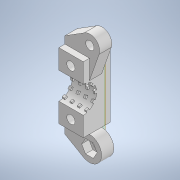
# Autodesk Inventor part: Rear Cable Clamp
Saved by Autodesk Inventor 2020 (Build 240168000, 168)
## iProperties
Created: 2019-12-14
Part Number: Rear Cable Clamp
Material: Generic
Document SubType Name: Modeling
Designer: pepd9
Density: 1 g/cm^3
Appearance: Default
Author: pepd9
Autodesk Inventor part; units mm, degrees
ref_plane "YZ Plane" through (0, 0, 0) normal (1, 0, 0) x (0, 1, 0)
ref_plane "XZ Plane" through (0, 0, 0) normal (0, 1, 0) x (-1, 0, 0)
ref_plane "XY Plane" through (0, 0, 0) normal (0, 0, 1) x (1, 0, 0)
sketch "Sketch1" plane through (0, 0, 0) normal (0, 0, 1) x (1, 0, 0)
  circle A0 centre (0, 0) radius 1.7
  circle A1 centre (0, 0) radius 5
  line L0 (0, 7) -> (0, -7) projected
  dimension "d0" = 10
  dimension "d6" = 3.4
  constraints: 2 centre point, 1 coincident
  measures "d0" diameter of A1
  measures "d6" diameter of A0
extrude "Extrusion1" add sketch "Sketch1" along normal blind 5 contours A0 L0 A1 | A0 L0 A1
sketch "Sketch2" plane through (0, 0, 5) normal (0, 0, 1) x (1, 0, 0)
  circle A0 centre (0, 0) radius 1.7 projected
  line L0 (1.5877, 2.75) -> (3.1754, 0)
  line L1 (3.1754, 0) -> (1.5877, -2.75)
  line L2 (1.5877, -2.75) -> (-1.5877, -2.75)
  line L3 (-1.5877, -2.75) -> (-3.1754, 0)
  line L4 (-3.1754, 0) -> (-1.5877, 2.75)
  line L5 (-1.5877, 2.75) -> (1.5877, 2.75)
  dimension "d3" = 5.5
  constraints: 12 end point, 1 coincident, 1 horizontal, 13 other
  measures "d3" distance between parallel lines of L2 L5
extrude "Extrusion2" cut sketch "Sketch2" against normal blind 3
sketch "Sketch3" plane through (0, 0, 0) normal (0, 0, -1) x (-1, 0, 0)
  point P0 (0, 0)
sketch "Sketch4" plane through (0, 0, 0) normal (1, 0, 0) x (0, 1, 0)
  line L0 (5, 0) -> (5, 5) projected
  line L1 (5, -3.5) -> (32, -3.5)
  line L2 (32, -3.5) -> (32, 7.5)
  line L3 (32, 7.5) -> (5, 7.5)
  line L4 (5, 7.5) -> (5, -3.5)
  circle A0 centre (18.5, 7.5) radius 5.5
  line L5 (5, 5) -> (-5, 5) projected
  point P0 (0, 0)
  point P1 (24, 7.5)
  point P2 (13, 7.5)
  dimension "d7" = 11
  dimension "d8" = 27
  dimension "d9" = 13.5
  dimension "d12" = 2.5
  dimension "d13" = 11
  constraints: 8 end point, 2 parallel, 1 centre point, 1 horizontal, 1 midpoint, 1 perpendicular, 1 point on line
  measures "d7" diameter of A0
  measures "d8" distance of L1.start L1.end
  measures "d9" distance from line of L4 A0.centre
  measures "d12" distance between parallel lines of L5 L3
  measures "d13" distance from line of L1 A0.centre
extrude "Extrusion3" add sketch "Sketch4" against normal blind 10 contours L0 L4 L3 A0 L2 L1
sketch "Sketch5" plane through (0, 0, 5) normal (0, 0, 1) x (1, 0, 0)
  circle A0 centre (0, 0) radius 5 projected
  line L0 (0, 5) -> (-10, 5) projected
  line L1 (0, 5) -> (-10, 5) projected
  line L2 (-10, 5) -> (-10, 0)
  line L3 (-10, 0) -> (-2.5, -4.3301)
  circle A1 centre (0, 0) radius 5 projected
  dimension "d30" = 5
  constraints: 4 end point, 1 point on circle, 1 tangent, 1 vertical, 1 other
  measures "d30" distance of L0.end L2.end
extrude "Extrusion4" add sketch "Sketch5" against normal up to surface (5 mm away) contours A0 L3 L2 L0
sketch "Sketch6" plane through (0, 5, -3.5) normal (0, 0, -1) x (-1, 0, 0)
  line L0 (0, 27) -> (10, 27) projected
  line L1 (0, 0) -> (10, 0) projected
  point P0 (0, -5)
  point P1 (5.0911, 4)
  point P2 (5.0911, 23)
  dimension "d16" = 4
  dimension "d17" = 4
  measures "d16" distance from line of L0 point (5.091, 23)
  measures "d17" distance from line of L1 point (5.091, 4)
hole "Hole1" at (-5.0911, 9, -3.5) at (-5.0911, 28, -3.5) direction (0, 0, 1) diameter 3.4 end through all counterbore diameter 6.5 counterbore depth 3 clearance for "Socket Head Cap Screw" size "M3" standard "Ansi Metric M Profile"
ref_plane "Work Plane1" through (0, 5, -1) normal (0, 0, -1) x (-1, 0, 0)
sketch "Sketch7" plane through (0, 5, -1) normal (0, 0, -1) x (-1, 0, 0)
  circle A0 centre (-0.2084, 31.6837) radius 1.7 projected
  circle A1 centre (-0.2084, 31.6837) radius 4
  line L0 (0, 19) -> (-3.9831, 30.3602)
  line L1 (0, 27) -> (10, 27) projected
  line L2 (0, 27) -> (0, 19) projected
  line L3 (10, 27) -> (10, 30)
  line L4 (10, 30) -> (2.0841, 34.9616)
  point P0 (0, -5)
  dimension "d26" = 8
  dimension "d27" = 3
  constraints: 6 end point, 2 point on circle, 1 centre point, 1 coincident, 1 tangent, 1 vertical
  measures "d26" diameter of A1
  measures "d27" distance of L1.end L3.end
extrude "Extrusion5" add sketch "Sketch7" against normal blind 5
sketch "Sketch8" plane through (-10, 0, 0) normal (-1, 0, 0) x (0, 0, 1)
  line L0 (7.5, 24) -> (7.5, 32) projected
  line L1 (7.5, 32) -> (4, 32) projected
  line L2 (4, 35) -> (4, 32) projected
  line L3 (-1, 35) -> (4, 35) projected
  line L4 (-1, 32) -> (-1, 35) projected
  line L5 (-1, 32) -> (-3.5, 32) projected
  line L6 (-3.5, 32) -> (-3.5, 5) projected
  line L7 (-3.5, 5) -> (0, 5) projected
  line L8 (0, 0) -> (0, 5) projected
  line L9 (5, 0) -> (0, 0) projected
  line L10 (5, 5) -> (5, 0) projected
  line L11 (5, 5) -> (7.5, 5) projected
  line L12 (7.5, 5) -> (7.5, 13) projected
  arc A0 (7.5, 24) -> (7.5, 13) centre (7.5, 18.5) ccw projected
  line L13 (7.5, 18.5) -> (6.2795, 24.2419)
  line L14 (7.5, 18.5) -> (5.0111, 24.0902)
  circle A1 centre (7.5, 18.5) radius 4.75
  point P0 (5.568, 22.8393)
  point P1 (6.5124, 23.1462)
  point P2 (6.3565, 23.8798)
  point P3 (5.2629, 23.5245)
  dimension "d31" = 12
  dimension "d32" = 12
  dimension "d33" = 9.5
  constraints: 4 end point, 1 centre point, 1 coincident
  measures "d31" angle of L0 L13
  measures "d32" angle of L13 L14
  measures "d33" diameter of A1
extrude "Extrusion6" add sketch "Sketch8" against normal blind 1 contours L13 A1 L14 A0
pattern_circular "Circular Pattern1" count 5 over 140 about axis through (0, 18.5, 7.5) along (-1, 0, 0) of "Extrusion6"
pattern_linear "Rectangular Pattern1" count 4 spacing 3 along (1, 0, 0) of "Extrusion6", "Circular Pattern1"
chamfer "Chamfer1" distance 0.25 distance2 0.75 1 edges at (-7, 23.0175, 6.0322) measured on face at (-6.5, 23.0175, 6.0322)
chamfer "Chamfer2" distance 0.25 distance2 0.75 1 edges at (-7, 21.3586, 3.7065) measured on face at (-6.5, 21.3586, 3.7065)
chamfer "Chamfer3" distance 0.25 distance2 0.75 1 edges at (-7, 18.6658, 2.7529) measured on face at (-6.5, 18.6658, 2.7529)
chamfer "Chamfer4" distance 0.25 distance2 0.75 1 edges at (-7, 15.913, 3.5163) measured on face at (-6.5, 15.913, 3.5163)
chamfer "Chamfer5" distance 0.25 distance2 0.75 1 edges at (-7, 14.0959, 5.7206) measured on face at (-6.5, 14.0959, 5.7206)
chamfer "Chamfer6" distance 0.25 distance2 0.75 1 edges at (-4, 14.0959, 5.7206) measured on face at (-3.5, 14.0959, 5.7206)
chamfer "Chamfer7" distance 0.25 distance2 0.75 1 edges at (-4, 15.913, 3.5163) measured on face at (-3.5, 15.913, 3.5163)
chamfer "Chamfer8" distance 0.25 distance2 0.75 1 edges at (-4, 18.6658, 2.7529) measured on face at (-3.5, 18.6658, 2.7529)
chamfer "Chamfer9" distance 0.25 distance2 0.75 1 edges at (-4, 21.3586, 3.7065) measured on face at (-3.5, 21.3586, 3.7065)
chamfer "Chamfer10" distance 0.25 distance2 0.75 1 edges at (-4, 23.0175, 6.0322) measured on face at (-3.5, 23.0175, 6.0322)
chamfer "Chamfer11" distance 0.25 distance2 0.75 1 edges at (-1, 23.0175, 6.0322) measured on face at (-0.5, 23.0175, 6.0322)
chamfer "Chamfer12" distance 0.25 distance2 0.75 1 edges at (-1, 21.3586, 3.7065) measured on face at (-0.5, 21.3586, 3.7065)
chamfer "Chamfer13" distance 0.25 distance2 0.75 1 edges at (-1, 18.6658, 2.7529) measured on face at (-0.5, 18.6658, 2.7529)
chamfer "Chamfer14" distance 0.25 distance2 0.75 1 edges at (-1, 15.913, 3.5163) measured on face at (-0.5, 15.913, 3.5163)
chamfer "Chamfer15" distance 0.25 distance2 0.75 1 edges at (-1, 14.0959, 5.7206) measured on face at (-0.5, 14.0959, 5.7206)
move faces "Move1" translate (0, 0, 1) faces at (-3.688, 33.1855, -1)
move faces "Move2" translate (0, 0, 1.5) faces at (-3.688, 33.1855, 4)
body "Solid1"
